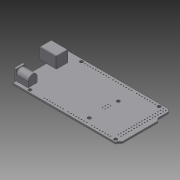
# Autodesk Inventor part: Arduino_Mega2560_R3
Saved by Autodesk Inventor 2014 (Build 180170000, 170)
## iProperties
Created: 2014-11-10
Part Number: Arduino_Mega2560_R3
Material: Generic
Document SubType Name: Modeling
Designer: ThatOtherGuy
Density: 1 g/cm^3
Appearance: Default
Author: ThatOtherGuy
Autodesk Inventor part; units mm, degrees
ref_plane "YZ Plane" through (0, 0, 0) normal (1, 0, 0) x (0, 1, 0)
ref_plane "XZ Plane" through (0, 0, 0) normal (0, 1, 0) x (-1, 0, 0)
ref_plane "XY Plane" through (0, 0, 0) normal (0, 0, 1) x (1, 0, 0)
sketch "Sketch1" plane through (0, 0, 0) normal (0, 0, 1) x (1, 0, 0)
  line L0 (0, 0) -> (99.06, 0)
  line L1 (99.06, 0) -> (99.06, 1.27)
  line L2 (99.06, 1.27) -> (101.6, 3.81)
  line L3 (101.6, 3.81) -> (101.6, 38.1)
  line L4 (101.6, 38.1) -> (99.06, 40.64)
  line L5 (99.06, 40.64) -> (99.06, 50.8)
  line L6 (99.06, 50.8) -> (96.52, 53.34)
  line L7 (96.52, 53.34) -> (0, 53.34)
  line L8 (0, 53.34) -> (0, 0)
  dimension "d1" = 1.27
  dimension "d2" = 53.34
  dimension "d3" = 101.6
  dimension "d4" = 99.06
  dimension "d5" = 45
  dimension "d6" = 38.1
  dimension "d7" = 2.54
  constraints: 18 end point, 4 perpendicular, 3 parallel, 1 collinear, 1 horizontal
  measures "d1" distance of L0.end L1.end
  measures "d2" distance of L7.end L0.start
  measures "d3" distance between parallel lines of L8 L3
  measures "d4" distance of L0.start L0.end
  measures "d5" angle of L5 L4
  measures "d6" distance from line of L3.end L0
  measures "d7" distance from line of L6.end L5
extrude "Board" add sketch "Sketch1" along normal blind 1.6
sketch "Sketch2" plane through (0, 0, 1.6) normal (0, 0, 1) x (1, 0, 0)
  line L0 (0, 53.34) -> (0, 0) projected
  line L1 (0, 0) -> (99.06, 0) projected
  point P0 (15.24, 50.8)
  point P1 (13.97, 2.54)
  point P2 (96.52, 2.54)
  point P3 (90.17, 50.8)
  point P4 (66.04, 35.56)
  point P5 (66.04, 7.62)
  dimension "d10" = 2.54
  dimension "d11" = 13.97
  dimension "d12" = 15.24
  dimension "d13" = 50.8
  dimension "d14" = 66.04
  dimension "d15" = 35.56
  dimension "d16" = 7.62
  dimension "d17" = 90.17
  dimension "d18" = 50.8
  dimension "d20" = 96.52
  constraints: 1 horizontal alignment, 1 vertical alignment
  measures "d10" vertical distance of L0.end point (13.97, 2.54)
  measures "d11" horizontal distance of point (13.97, 2.54) L0.end
  measures "d12" distance from line of L0 point (15.24, 50.8)
  measures "d13" vertical distance of L0.end point (15.24, 50.8)
  measures "d14" distance from line of L0 point (66.04, 35.56)
  measures "d15" vertical distance of L0.end point (66.04, 35.56)
  measures "d16" distance from line of L1 point (66.04, 7.62)
  measures "d17" horizontal distance of L0.end point (90.17, 50.8)
  measures "d18" distance from line of L1 point (90.17, 50.8)
  measures "d20" horizontal distance of L0.end point (96.52, 2.54)
hole "Mounting Holes" at (15.24, 50.8, 1.6) at (13.97, 2.54, 1.6) at (96.52, 2.54, 1.6) at (90.17, 50.8, 1.6) at (66.04, 35.56, 1.6) at (66.04, 7.62, 1.6) direction (0, 0, -1) diameter 3.175 end through all
sketch "Sketch3" plane through (0, 0, 1.6) normal (0, 0, 1) x (1, 0, 0)
  line L0 (0, 53.34) -> (0, 0) projected
  line L1 (0, 0) -> (99.06, 0) projected
  line L2 (-1.905, 3.175) -> (11.43, 3.175)
  line L3 (11.43, 3.175) -> (11.43, 12.065)
  line L4 (11.43, 12.065) -> (-1.905, 12.065)
  line L5 (-1.905, 3.175) -> (-1.905, 12.065)
  dimension "d28" = 3.175
  dimension "d29" = 12.065
  dimension "d30" = 11.43
  dimension "d159" = 1.905
  constraints: 8 end point, 2 perpendicular, 1 horizontal, 1 parallel
  measures "d28" distance between parallel lines of L1 L2
  measures "d29" distance between parallel lines of L1 L4
  measures "d30" distance from line of L0.end L3
  measures "d159" distance between parallel lines of L0 L5
extrude "PowerJack" add sketch "Sketch3" along normal blind 10
sketch "Sketch7" plane through (11.43, 3.175, 1.6) normal (1, 0, 0) x (0, 0, -1)
  line L0 (0, 8.89) -> (0, 0) projected
  line L1 (0, 8.89) -> (-10, 8.89) projected
  line L2 (-10, 0) -> (-10, 8.89) projected
  line L3 (0, 0) -> (-10, 0) projected
  arc A0 (-5.055, 8.89) -> (-5.055, 0) centre (-5.055, 4.445) ccw
  point P0 (1.6, -3.175)
  dimension "d177" = 0.5
  constraints: 2 point on circle, 2 point on line, 2 tangent, 1 centre point
  measures "d177" distance edge to line of A0 L2
extrude "PowerJack_Barrel" cut sketch "Sketch7" against normal blind 11.43 contours A0 L3 L2 L1
sketch "Sketch14" plane through (-1.905, 3.175, 1.6) normal (-1, 0, 0) x (0, 0, 1)
  line L0 (10, 8.89) -> (10, 0) projected
  circle A0 centre (5, 4.445) radius 3
  point P0 (-1.6, -3.175)
  point P1 (10, 4.445)
  dimension "d194" = 2
  dimension "d195" = 6
  constraints: 1 centre point, 1 horizontal alignment, 1 midpoint
  measures "d194" distance edge to line of A0 L0
  measures "d195" diameter of A0
extrude "PowerJack_Inset" cut sketch "Sketch14" against normal blind 10
sketch "Sketch15" plane through (8.095, 7.62, 6.6) normal (-1, 0, 0) x (0, 0, 1)
  circle A0 centre (0, 0) radius 3 projected
  circle A1 centre (0, 0) radius 1.25
  point P0 (-6.6, -7.62)
  dimension "d198" = 2.5
  constraints: 1 centre point, 1 coincident
  measures "d198" diameter of A1
extrude "PowerJack_Pin" add sketch "Sketch15" along normal blind 8 contours A1
sketch "Sketch4" plane through (0, 0, 1.6) normal (0, 0, 1) x (1, 0, 0)
  line L0 (0, 53.34) -> (0, 0) projected
  line L1 (-6.35, 43.815) -> (9.525, 43.815)
  line L2 (9.525, 43.815) -> (9.525, 32.385)
  line L3 (9.525, 32.385) -> (-6.35, 32.385)
  line L4 (11.43, 12.065) -> (11.43, 3.175) projected
  line L5 (-6.35, 43.815) -> (-6.35, 32.385)
  dimension "d33" = 32.385
  dimension "d34" = 43.815
  dimension "d35" = 9.525
  dimension "d160" = 6.35
  constraints: 8 end point, 2 parallel, 1 horizontal, 1 perpendicular
  measures "d33" distance from line of L0.end L3
  measures "d34" distance from line of L0.end L1
  measures "d35" distance between parallel lines of L0 L2
  measures "d160" distance between parallel lines of L0 L5
extrude "USBJack" add sketch "Sketch4" along normal blind 10.795
sketch "Sketch13" plane through (-6.35, 32.385, 1.6) normal (-1, 0, 0) x (0, 0, 1)
  line L0 (0, 0) -> (0, 11.43) projected
  line L1 (0, 0) -> (10.795, 0) projected
  line L2 (10.795, 11.43) -> (10.795, 0) projected
  line L3 (0, 11.43) -> (10.795, 11.43) projected
  line L4 (2, 9.43) -> (7.295, 9.43)
  line L5 (8.795, 7.93) -> (8.795, 3.5)
  line L6 (7.295, 2) -> (2, 2)
  line L7 (2, 2) -> (2, 9.43)
  line L8 (7.295, 9.43) -> (8.795, 7.93)
  line L9 (8.795, 3.5) -> (7.295, 2)
  line L10 (4.3975, 7.215) -> (6.3975, 7.215)
  line L11 (6.3975, 7.215) -> (6.3975, 4.215)
  line L12 (6.3975, 4.215) -> (4.3975, 4.215)
  line L13 (4.3975, 4.215) -> (4.3975, 7.215)
  point P0 (-1.6, -32.385)
  point P1 (2, 5.715)
  point P2 (4.3975, 5.715)
  dimension "d182" = 1.5
  dimension "d183" = 45
  dimension "d184" = 2
  dimension "d185" = 3
  dimension "d186" = 2.3975
  dimension "d187" = 2.3975
  dimension "d188" = 2
  dimension "d189" = 2
  dimension "d190" = 2
  dimension "d191" = 2
  constraints: 20 end point, 4 parallel, 4 perpendicular, 2 horizontal, 2 midpoint, 1 horizontal alignment
  measures "d182" horizontal distance of L6.start L5.end
  measures "d183" angle of L5 L9
  measures "d184" distance of L13.end L11.start
  measures "d185" distance of L13.start L13.end
  measures "d186" distance between parallel lines of L7 L13
  measures "d187" distance between parallel lines of L5 L11
  measures "d188" distance between parallel lines of L3 L4
  measures "d189" distance between parallel lines of L1 L6
  measures "d190" distance between parallel lines of L0 L7
  measures "d191" distance between parallel lines of L2 L5
extrude "USBJack_Inset" cut sketch "Sketch13" against normal blind 10 contours L4 L8 L5 L9 L6 L7
fillet "PowerUSBFillet" radius 0.5 10 edges at (1.5875, 32.385, 12.395) (1.5875, 43.815, 12.395) (-0.9525, 3.175, 11.6) (-0.9525, 12.065, 11.6) (9.525, 38.1, 12.395) (9.525, 32.385, 6.9975) (9.525, 43.815, 6.9975) (0, 7.62, 11.1) (-3.175, 32.385, 1.6) (-3.175, 43.815, 1.6)
sketch "Sketch9" plane through (0, 0, 1.6) normal (0, 0, 1) x (1, 0, 0)
  line L0 (0, 53.34) -> (0, 0) projected
  line L1 (0, 0) -> (99.06, 0) projected
  line L2 (96.52, 53.34) -> (0, 53.34) projected
  point P0 (93.98, 7.62)
  point P1 (27.94, 2.54)
  point P2 (50.8, 2.54)
  point P3 (73.66, 2.54)
  point P4 (18.796, 50.8)
  point P5 (45.72, 50.8)
  point P6 (68.58, 50.8)
  point P7 (21.336, 50.8)
  point P8 (23.876, 50.8)
  point P9 (26.416, 50.8)
  point P10 (28.956, 50.8)
  point P11 (31.496, 50.8)
  point P12 (34.036, 50.8)
  point P13 (36.576, 50.8)
  point P14 (39.116, 50.8)
  point P15 (41.656, 50.8)
  point P16 (96.52, 7.62)
  point P17 (93.98, 10.16)
  point P18 (96.52, 10.16)
  point P19 (93.98, 12.7)
  point P20 (96.52, 12.7)
  point P21 (93.98, 15.24)
  point P22 (96.52, 15.24)
  point P23 (93.98, 17.78)
  point P24 (96.52, 17.78)
  point P25 (93.98, 20.32)
  point P26 (96.52, 20.32)
  point P27 (93.98, 22.86)
  point P28 (96.52, 22.86)
  point P29 (93.98, 25.4)
  point P30 (96.52, 25.4)
  point P31 (93.98, 27.94)
  point P32 (96.52, 27.94)
  point P33 (93.98, 30.48)
  point P34 (96.52, 30.48)
  point P35 (93.98, 33.02)
  point P36 (96.52, 33.02)
  point P37 (93.98, 35.56)
  point P38 (96.52, 35.56)
  point P39 (93.98, 38.1)
  point P40 (96.52, 38.1)
  point P41 (93.98, 40.64)
  point P42 (96.52, 40.64)
  point P43 (93.98, 43.18)
  point P44 (96.52, 43.18)
  point P45 (93.98, 45.72)
  point P46 (96.52, 45.72)
  point P47 (93.98, 48.26)
  point P48 (96.52, 48.26)
  point P49 (93.98, 50.8)
  point P50 (96.52, 50.8)
  point P51 (30.48, 2.54)
  point P52 (53.34, 2.54)
  point P53 (76.2, 2.54)
  point P54 (48.26, 50.8)
  point P55 (71.12, 50.8)
  point P56 (33.02, 2.54)
  point P57 (55.88, 2.54)
  point P58 (78.74, 2.54)
  point P59 (50.8, 50.8)
  point P60 (73.66, 50.8)
  point P61 (35.56, 2.54)
  point P62 (58.42, 2.54)
  point P63 (81.28, 2.54)
  point P64 (53.34, 50.8)
  point P65 (76.2, 50.8)
  point P66 (38.1, 2.54)
  point P67 (60.96, 2.54)
  point P68 (83.82, 2.54)
  point P69 (55.88, 50.8)
  point P70 (78.74, 50.8)
  point P71 (40.64, 2.54)
  point P72 (63.5, 2.54)
  point P73 (86.36, 2.54)
  point P74 (58.42, 50.8)
  point P75 (81.28, 50.8)
  point P76 (43.18, 2.54)
  point P77 (66.04, 2.54)
  point P78 (88.9, 2.54)
  point P79 (60.96, 50.8)
  point P80 (83.82, 50.8)
  point P81 (45.72, 2.54)
  point P82 (68.58, 2.54)
  point P83 (91.44, 2.54)
  point P84 (63.5, 50.8)
  point P85 (86.36, 50.8)
  dimension "d103" = 2.54
  dimension "d104" = 27.94
  dimension "d105" = 50.8
  dimension "d106" = 73.66
  dimension "d107" = 93.98
  dimension "d108" = 7.62
  dimension "d109" = 50.8
  dimension "d110" = 18.796
  dimension "d111" = 45.72
  dimension "d112" = 68.58
  dimension "d115" = 2.54
  dimension "d122" = 2.54
  dimension "d125" = 2.54
  dimension "d130" = 2.54
  constraints: 4 horizontal alignment, 3 horizontal, 1 vertical, 79 other
  measures "d103" distance from line of L1 point (27.94, 2.54)
  measures "d104" distance from line of L0 point (27.94, 2.54)
  measures "d105" distance from line of L0 point (50.8, 2.54)
  measures "d106" distance from line of L0 point (73.66, 2.54)
  measures "d107" distance from line of L0 point (93.98, 7.62)
  measures "d108" distance from line of L1 point (93.98, 7.62)
  measures "d109" distance from line of L1 point (18.796, 50.8)
  measures "d110" distance from line of L0 point (18.796, 50.8)
  measures "d111" distance from line of L0 point (45.72, 50.8)
  measures "d112" distance from line of L0 point (68.58, 50.8)
  measures "d115" distance of point (18.796, 50.8) point (21.336, 50.8)
  measures "d122" distance of point (93.98, 7.62) point (96.52, 7.62)
  measures "d125" distance of point (93.98, 7.62) point (93.98, 10.16)
  measures "d130" distance of point (45.72, 50.8) point (48.26, 50.8)
hole "Header_Holes" at (93.98, 7.62, 1.6) at (27.94, 2.54, 1.6) at (50.8, 2.54, 1.6) at (73.66, 2.54, 1.6) at (18.796, 50.8, 1.6) at (45.72, 50.8, 1.6) at (68.58, 50.8, 1.6) at (21.336, 50.8, 1.6) at (23.876, 50.8, 1.6) at (26.416, 50.8, 1.6) at (28.956, 50.8, 1.6) at (31.496, 50.8, 1.6) at (34.036, 50.8, 1.6) at (36.576, 50.8, 1.6) at (39.116, 50.8, 1.6) at (41.656, 50.8, 1.6) at (96.52, 7.62, 1.6) at (93.98, 10.16, 1.6) at (96.52, 10.16, 1.6) at (93.98, 12.7, 1.6) at (96.52, 12.7, 1.6) at (93.98, 15.24, 1.6) at (96.52, 15.24, 1.6) at (93.98, 17.78, 1.6) at (96.52, 17.78, 1.6) at (93.98, 20.32, 1.6) at (96.52, 20.32, 1.6) at (93.98, 22.86, 1.6) at (96.52, 22.86, 1.6) at (93.98, 25.4, 1.6) at (96.52, 25.4, 1.6) at (93.98, 27.94, 1.6) at (96.52, 27.94, 1.6) at (93.98, 30.48, 1.6) at (96.52, 30.48, 1.6) at (93.98, 33.02, 1.6) at (96.52, 33.02, 1.6) at (93.98, 35.56, 1.6) at (96.52, 35.56, 1.6) at (93.98, 38.1, 1.6) at (96.52, 38.1, 1.6) at (93.98, 40.64, 1.6) at (96.52, 40.64, 1.6) at (93.98, 43.18, 1.6) at (96.52, 43.18, 1.6) at (93.98, 45.72, 1.6) at (96.52, 45.72, 1.6) at (93.98, 48.26, 1.6) at (96.52, 48.26, 1.6) at (93.98, 50.8, 1.6) direction (0, 0, -1) diameter 0.889 end through all and at (96.52, 50.8, 1.6) (48.26, 50.8, 1.6) (71.12, 50.8, 1.6) (76.2, 2.54, 1.6) (53.34, 2.54, 1.6) (30.48, 2.54, 1.6) (50.8, 50.8, 1.6) (73.66, 50.8, 1.6) (78.74, 2.54, 1.6) (55.88, 2.54, 1.6) (33.02, 2.54, 1.6) (53.34, 50.8, 1.6) (76.2, 50.8, 1.6) (81.28, 2.54, 1.6) (58.42, 2.54, 1.6) (35.56, 2.54, 1.6) (55.88, 50.8, 1.6) (78.74, 50.8, 1.6) (83.82, 2.54, 1.6) (60.96, 2.54, 1.6) (38.1, 2.54, 1.6) (58.42, 50.8, 1.6) (81.28, 50.8, 1.6) (86.36, 2.54, 1.6) (63.5, 2.54, 1.6) (40.64, 2.54, 1.6) (60.96, 50.8, 1.6) (83.82, 50.8, 1.6) (88.9, 2.54, 1.6) (66.04, 2.54, 1.6) (43.18, 2.54, 1.6) (63.5, 50.8, 1.6) (86.36, 50.8, 1.6) (91.44, 2.54, 1.6) (68.58, 2.54, 1.6) (45.72, 2.54, 1.6)
sketch "Sketch10" plane through (0, 0, 1.6) normal (0, 0, 1) x (1, 0, 0)
  line L0 (0, 53.34) -> (0, 0) projected
  line L1 (0, 0) -> (99.06, 0) projected
  line L2 (101.6, 3.81) -> (101.6, 38.1) projected
  point P0 (63.627, 27.94)
  point P1 (63.627, 25.4)
  point P2 (63.627, 22.86)
  point P3 (66.167, 27.94)
  point P4 (66.167, 25.4)
  point P5 (66.167, 22.86)
  dimension "d142" = 63.627
  dimension "d143" = 27.94
  dimension "d146" = 2.54
  dimension "d149" = 2.54
  constraints: 1 horizontal, 1 vertical, 5 other
  measures "d142" distance from line of L0 point (63.627, 27.94)
  measures "d143" distance from line of point (63.627, 27.94) L1
  measures "d146" distance of point (63.627, 27.94) point (63.627, 25.4)
  measures "d149" distance of point (63.627, 27.94) point (66.167, 27.94)
hole "ICSP_Header_Holes" at (63.627, 27.94, 1.6) at (63.627, 25.4, 1.6) at (63.627, 22.86, 1.6) at (66.167, 27.94, 1.6) at (66.167, 25.4, 1.6) at (66.167, 22.86, 1.6) direction (0, 0, -1) diameter 0.889 end through all
equation "\"d186\" = d187"
equation "\"d189\" = d188"
equation "\"d190\" = d188"
equation "\"d191\" = d190"
body "Solid1"
